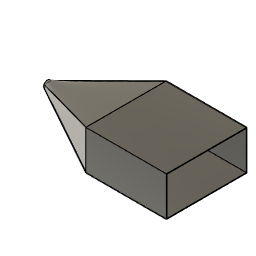
small aperture reactor 1 v1 (Autodesk Fusion 360 design; units mm, degrees)
Autodesk Fusion 360 part; units mm, degrees
note: some values were not read from the file. Chosen so that the rebuilt part matches the saved one: which face or edge a step refers to.
sketch "Sketch1" plane through (0, 0, 0) normal (0, 0, 1) x (1, 0, 0)
  line L0 (0, 0) -> (210, 0)
  line L1 (210, 0) -> (210, 210)
  line L2 (210, 210) -> (0, 210)
  line L3 (0, 210) -> (0, 0)
  dimension "d1" = 210
  dimension "d2" = 210
  constraint horizontal L0
  constraint vertical L1
  constraint horizontal L2
  constraint vertical L3
  constraint coincident L0.start L3.end
  measures "d1" distance of L0.start L0.end
  measures "d2" distance of L0.start L2.end
extrude "Extrude1" add sketch "Sketch1" along normal blind 103
shell "Shell1" thickness 1.5 removed faces 1 at (0, 140, 68.6667)
delete_face "DeleteFace1" 2 faces at (210, 70, 68.6667) (208.5, 139.5, 68.1667)
sketch "Sketch2" plane through (0, 0, 0) normal (1, 0, 0) x (0, 1, 0)
  line L0 (0, 0) -> (210, 0)
  line L1 (210, 0) -> (210, 103)
  line L2 (210, 103) -> (0, 103)
  line L3 (0, 103) -> (0, 0)
  constraint horizontal L0
  constraint vertical L1
  constraint horizontal L2
  constraint vertical L3
  constraint coincident L0.start L3.end
sketch "Sketch3" plane through (0, 0, 0) normal (1, 0, 0) x (0, 1, 0)
  circle A0 centre (100, 50) radius 10
  dimension "d6" = 20
  measures "d6" diameter of A0
sketch "Sketch4" plane through (-200, 0, 0) normal (-1, 0, 0) x (0, -1, 0)
  circle A0 centre (-100, 50) radius 10
  circle A1 centre (-100, 50) radius 10
  constraint concentric A0 A1
loft "Loft1" add profiles "Sketch4", "Sketch2" section 1 section 2
shell "Shell2" thickness 1.5 removed faces 1 at (0, 139.5, 34.8333)
sketch "Sketch5" plane through (-200, 0, 0) normal (-1, 0, 0) x (0, -1, 0)
  arc A0 (-91.0218, 54.4036) -> (-108.9782, 54.4036) centre (-100, 50) ccw
  arc A1 (-108.9782, 54.4036) -> (-108.9782, 45.5964) centre (-100, 50) ccw
  arc A2 (-108.9782, 45.5964) -> (-91.0218, 45.5964) centre (-100, 50) ccw
  arc A3 (-91.0218, 45.5964) -> (-91.0218, 54.4036) centre (-100, 50) ccw
  line L0 (-100, 50) -> (-100, 40)
  constraint coincident A0.centre A1.centre
  constraint midpoint A2 L0.end
hole "Hole1" at (-200, 100, 50) direction (1, 0, 0) diameter 20 depth 45 tip angle 118
